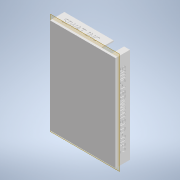
# Autodesk Inventor part: Buttom Plate
Saved by Autodesk Inventor 2020 (Build 240168000, 168)
## iProperties
Created: 2019-11-08
Part Number: Buttom Plate
Material: Generic
Document SubType Name: Modeling
Designer: siwat
Density: 1 g/cm^3
Appearance: Default
Author: siwat
Autodesk Inventor part; units mm, degrees
ref_plane "YZ Plane" through (0, 0, 0) normal (1, 0, 0) x (0, 1, 0)
ref_plane "XZ Plane" through (0, 0, 0) normal (0, 1, 0) x (-1, 0, 0)
ref_plane "XY Plane" through (0, 0, 0) normal (0, 0, 1) x (1, 0, 0)
ref_plane "Work Plane1" through (0, 0, 0) normal (0, 0, 1) x (1, 0, 0)
sketch "Sketch1" plane through (0, 0, 0) normal (0, 0, 1) x (1, 0, 0)
  line L0 (38.904, 56.6039) -> (-39.0955, 56.6039)
  line L1 (-39.0955, 56.6039) -> (-39.0955, -56.8569)
  line L2 (-39.0955, -56.8569) -> (38.904, -56.8569)
  line L3 (38.904, -56.8569) -> (38.904, 56.6039)
  line L4 (-37.4141, -55.0738) -> (37.4715, -55.0738)
  line L5 (37.4715, -55.0738) -> (37.4715, 55.1115)
  line L6 (37.4715, 55.1115) -> (-37.4141, 55.1115)
  line L7 (-37.4141, 55.1115) -> (-37.4141, -55.0738)
  point P0 (0, 0)
  constraints: 16 end point, 4 parallel, 2 horizontal, 2 perpendicular
extrude "Extrusion1" add sketch "Sketch1" along normal blind 2.0625 and the other way blind 14.525
sketch "Sketch2" plane through (0, 0, 2.0625) normal (0, 0, 1) x (1, 0, 0)
  line L0 (38.904, 56.6039) -> (-39.0955, 56.6039)
  line L1 (-39.0955, 56.6039) -> (-39.0955, -56.8569)
  line L2 (-39.0955, -56.8569) -> (38.904, -56.8569)
  line L3 (38.904, -56.8569) -> (38.904, 56.6039)
  point P0 (0, 0)
  constraints: 8 end point, 2 parallel, 1 horizontal, 1 perpendicular
extrude "Extrusion2" add sketch "Sketch2" along normal blind 0.59
sketch "Sketch3" plane through (-39.0955, -56.8569, -14.525) normal (-1, 0, 0) x (0, 0, 1)
  line L0 (14.525, 65.2907) -> (0, 65.2907)
  line L1 (0, 65.2907) -> (0, 84.283)
  line L2 (0, 84.283) -> (14.525, 84.283)
  line L3 (14.525, 84.283) -> (14.525, 65.2907)
  line L4 (0, 0) -> (0, 113.4608) projected
  point P0 (14.525, 56.8569)
  constraints: 8 end point, 2 parallel, 1 horizontal, 1 perpendicular, 1 point on line
extrude "Extrusion3" cut sketch "Sketch3" against normal up to surface (1.6814 mm away)
sketch "Sketch4" plane through (-39.0955, 56.6039, -14.525) normal (0, 1, 0) x (1, 0, 0)
  line L0 (77.9995, 0) -> (0, 0) projected
  line L1 (58.5885, -14.525) -> (71.0413, -14.525)
  line L2 (71.0413, -14.525) -> (71.0413, 0)
  line L3 (71.0413, 0) -> (58.5885, 0)
  line L4 (58.5885, 0) -> (58.5885, -14.525)
  point P0 (39.0955, -14.525)
  constraints: 8 end point, 2 parallel, 1 horizontal, 1 perpendicular, 1 point on line
extrude "Extrusion4" cut sketch "Sketch4" against normal up to surface (1.4924 mm away)
sketch "Sketch6" plane through (0, 0, 2.0625) normal (0, 0, -1) x (-1, 0, 0)
  line L0 (35.9141, -53.5738) -> (-35.9715, -53.5738)
  line L1 (-35.9715, -53.5738) -> (-35.9715, 53.6115)
  line L2 (-35.9715, 53.6115) -> (35.9141, 53.6115)
  line L3 (35.9141, 53.6115) -> (35.9141, -53.5738)
  line L4 (-37.4715, 55.1115) -> (-31.9458, 55.1115) projected
  line L5 (-37.4715, -55.0738) -> (-37.4715, 55.1115) projected
  line L6 (37.4141, -55.0738) -> (-37.4715, -55.0738) projected
  line L7 (37.4141, 8.4338) -> (37.4141, -55.0738) projected
  line L8 (37.4141, -55.0738) -> (37.4141, 55.1115) projected
  line L9 (-37.4715, 55.1115) -> (-37.4715, -55.0738) projected
  line L10 (37.4141, -55.0738) -> (-37.4715, -55.0738)
  line L11 (-37.4715, -55.0738) -> (-37.4715, 55.1115)
  line L12 (-37.4715, 55.1115) -> (37.4141, 55.1115)
  line L13 (37.4141, 55.1115) -> (37.4141, -55.0738)
  point P0 (0, 0)
  dimension "d12" = 1.5
  dimension "d13" = 1.5
  dimension "d14" = 1.5
  dimension "d15" = 1.5
  constraints: 16 end point, 4 parallel, 2 horizontal, 2 perpendicular
  measures "d12" distance between parallel lines of L2 L4
  measures "d13" distance between parallel lines of L5 L1
  measures "d14" distance between parallel lines of L6 L0
  measures "d15" distance between parallel lines of L7 L3
extrude "Extrusion6" add sketch "Sketch6" along normal up to surface (2.0625 mm away)
sketch "Sketch5" plane through (0, 0, 2.0625) normal (0, 0, -1) x (-1, 0, 0)
  circle A0 centre (33.0429, -48.5316) radius 1.6001
  circle A1 centre (11.8743, 21.7468) radius 1.6087
  circle A2 centre (-29.2374, 31.3404) radius 1.6463
  circle A3 centre (-15.7576, -8.1834) radius 1.5639
  circle A4 centre (-29.803, -47.9298) radius 1.5995
  point P0 (0, 0)
  constraints: 5 centre point
extrude "Extrusion5" add sketch "Sketch5" along normal blind 4.5
sketch "Sketch7" plane through (-39.0955, 56.6039, 2.6525) normal (0, 1, 0) x (1, 0, 0)
  line L0 (6.9784, 11.7138) -> (55.3893, 11.7138) construction
  line L1 (55.3893, 11.7138) -> (55.3893, 4.2787) construction
  line L2 (55.3893, 4.2787) -> (6.9784, 4.2787) construction
  line L3 (6.9784, 4.2787) -> (6.9784, 11.7138) construction
  spline S0 degree 2 poles (9.2953, 5.4005) (8.6333, 5.4005) (7.7046, 5.6771) (7.2946, 5.8747) knots 0 0 0 1 2 2 2
  line L4 (7.2946, 5.8747) -> (7.2946, 6.8924)
  line L5 (7.2946, 6.8924) -> (7.3538, 6.8924)
  spline S1 degree 2 poles (7.3538, 6.8924) (7.754, 6.5169) (8.7667, 6.102) (9.236, 6.102) knots 0 0 0 1 2 2 2
  spline S2 degree 2 poles (9.236, 6.102) (9.9078, 6.102) (10.5945, 6.6602) (10.5945, 7.1196) knots 0 0 0 1 2 2 2
  spline S3 degree 2 poles (10.5945, 7.1196) (10.5945, 7.4852) (10.2339, 7.9396) (9.8436, 8.0533) knots 0 0 0 1 2 2 2
  spline S4 degree 2 poles (9.8436, 8.0533) (9.562, 8.1323) (9.0927, 8.241) (8.742, 8.3299) knots 0 0 0 1 2 2 2
  spline S5 degree 2 poles (8.742, 8.3299) (8.4258, 8.4139) (7.9269, 8.6658) (7.7342, 8.8684) knots 0 0 0 1 2 2 2
  spline S6 degree 2 poles (7.7342, 8.8684) (7.5465, 9.0709) (7.339, 9.6143) (7.339, 9.97) knots 0 0 0 1 2 2 2
  spline S7 degree 2 poles (7.339, 9.97) (7.339, 10.711) (8.495, 11.7138) (9.3891, 11.7138) knots 0 0 0 1 2 2 2
  spline S8 degree 2 poles (9.3891, 11.7138) (9.9029, 11.7138) (10.8119, 11.5113) (11.2021, 11.3186) knots 0 0 0 1 2 2 2
  line L6 (11.2021, 11.3186) -> (11.2021, 10.3504)
  line L7 (11.2021, 10.3504) -> (11.1429, 10.3504)
  spline S9 degree 2 poles (11.1429, 10.3504) (10.8514, 10.6171) (9.9424, 11.0123) (9.4435, 11.0123) knots 0 0 0 1 2 2 2
  spline S10 degree 2 poles (9.4435, 11.0123) (8.8803, 11.0123) (8.1838, 10.4838) (8.1838, 10.054) knots 0 0 0 1 2 2 2
  spline S11 degree 2 poles (8.1838, 10.054) (8.1838, 9.6687) (8.5938, 9.2092) (8.9791, 9.1055) knots 0 0 0 1 2 2 2
  spline S12 degree 2 poles (8.9791, 9.1055) (9.236, 9.0363) (9.9819, 8.8585) (10.2289, 8.7844) knots 0 0 0 1 2 2 2
  spline S13 degree 2 poles (10.2289, 8.7844) (10.8563, 8.5917) (11.4393, 7.8161) (11.4393, 7.248) knots 0 0 0 1 2 2 2
  spline S14 degree 2 poles (11.4393, 7.248) (11.4393, 6.8874) (11.1478, 6.1958) (10.886, 5.9537) knots 0 0 0 1 2 2 2
  spline S15 degree 2 poles (10.886, 5.9537) (10.5945, 5.687) (9.8535, 5.4005) (9.2953, 5.4005) knots 0 0 0 1 2 2 2
  line L8 (14.3885, 5.5091) -> (12.0271, 5.5091)
  line L9 (12.0271, 5.5091) -> (12.0271, 6.1316)
  line L10 (12.0271, 6.1316) -> (12.8027, 6.1316)
  line L11 (12.8027, 6.1316) -> (12.8027, 10.9827)
  line L12 (12.8027, 10.9827) -> (12.0271, 10.9827)
  line L13 (12.0271, 10.9827) -> (12.0271, 11.6051)
  line L14 (12.0271, 11.6051) -> (14.3885, 11.6051)
  line L15 (14.3885, 11.6051) -> (14.3885, 10.9827)
  line L16 (14.3885, 10.9827) -> (13.6129, 10.9827)
  line L17 (13.6129, 10.9827) -> (13.6129, 6.1316)
  line L18 (13.6129, 6.1316) -> (14.3885, 6.1316)
  line L19 (14.3885, 6.1316) -> (14.3885, 5.5091)
  line L20 (22.2233, 11.6051) -> (20.6919, 5.5091)
  line L21 (20.6919, 5.5091) -> (19.783, 5.5091)
  line L22 (19.783, 5.5091) -> (18.543, 10.5677)
  line L23 (18.543, 10.5677) -> (17.3377, 5.5091)
  line L24 (17.3377, 5.5091) -> (16.4386, 5.5091)
  line L25 (16.4386, 5.5091) -> (14.8825, 11.6051)
  line L26 (14.8825, 11.6051) -> (15.7173, 11.6051)
  line L27 (15.7173, 11.6051) -> (16.9425, 6.5515)
  line L28 (16.9425, 6.5515) -> (18.1577, 11.6051)
  line L29 (18.1577, 11.6051) -> (18.9827, 11.6051)
  line L30 (18.9827, 11.6051) -> (20.2078, 6.4922)
  line L31 (20.2078, 6.4922) -> (21.428, 11.6051)
  line L32 (21.428, 11.6051) -> (22.2233, 11.6051)
  line L33 (22.2925, 5.5091) -> (24.3476, 11.6051)
  line L34 (24.3476, 11.6051) -> (25.3454, 11.6051)
  line L35 (25.3454, 11.6051) -> (27.4005, 5.5091)
  line L36 (27.4005, 5.5091) -> (26.5459, 5.5091)
  line L37 (26.5459, 5.5091) -> (25.9926, 7.2135)
  line L38 (25.9926, 7.2135) -> (23.6658, 7.2135)
  line L39 (23.6658, 7.2135) -> (23.1126, 5.5091)
  line L40 (23.1126, 5.5091) -> (22.2925, 5.5091)
  line L41 (25.7703, 7.9051) -> (24.8267, 10.7752)
  line L42 (24.8267, 10.7752) -> (23.8881, 7.9051)
  line L43 (23.8881, 7.9051) -> (25.7703, 7.9051)
  line L44 (29.4012, 5.5091) -> (29.4012, 10.8839)
  line L45 (29.4012, 10.8839) -> (27.356, 10.8839)
  line L46 (27.356, 10.8839) -> (27.356, 11.6051)
  line L47 (27.356, 11.6051) -> (32.2566, 11.6051)
  line L48 (32.2566, 11.6051) -> (32.2566, 10.8839)
  line L49 (32.2566, 10.8839) -> (30.2114, 10.8839)
  line L50 (30.2114, 10.8839) -> (30.2114, 5.5091)
  line L51 (30.2114, 5.5091) -> (29.4012, 5.5091)
  line L52 (37.6165, 5.5091) -> (35.2552, 5.5091)
  line L53 (35.2552, 5.5091) -> (35.2552, 6.1316)
  line L54 (35.2552, 6.1316) -> (36.0307, 6.1316)
  line L55 (36.0307, 6.1316) -> (36.0307, 10.9827)
  line L56 (36.0307, 10.9827) -> (35.2552, 10.9827)
  line L57 (35.2552, 10.9827) -> (35.2552, 11.6051)
  line L58 (35.2552, 11.6051) -> (37.6165, 11.6051)
  line L59 (37.6165, 11.6051) -> (37.6165, 10.9827)
  line L60 (37.6165, 10.9827) -> (36.8409, 10.9827)
  line L61 (36.8409, 10.9827) -> (36.8409, 6.1316)
  line L62 (36.8409, 6.1316) -> (37.6165, 6.1316)
  line L63 (37.6165, 6.1316) -> (37.6165, 5.5091)
  line L64 (42.9814, 5.5091) -> (42.0724, 5.5091)
  line L65 (42.0724, 5.5091) -> (39.3751, 10.7653)
  line L66 (39.3751, 10.7653) -> (39.3751, 5.5091)
  line L67 (39.3751, 5.5091) -> (38.6193, 5.5091)
  line L68 (38.6193, 5.5091) -> (38.6193, 11.6051)
  line L69 (38.6193, 11.6051) -> (39.7703, 11.6051)
  line L70 (39.7703, 11.6051) -> (42.2255, 6.7787)
  line L71 (42.2255, 6.7787) -> (42.2255, 11.6051)
  line L72 (42.2255, 11.6051) -> (42.9814, 11.6051)
  line L73 (42.9814, 11.6051) -> (42.9814, 5.5091)
  spline S16 degree 2 poles (46.5975, 5.4005) (46.0047, 5.4005) (45.0018, 5.8006) (44.6363, 6.2008) knots 0 0 0 1 2 2 2
  spline S17 degree 2 poles (44.6363, 6.2008) (44.2707, 6.596) (43.8706, 7.7816) (43.8706, 8.5522) knots 0 0 0 1 2 2 2
  spline S18 degree 2 poles (43.8706, 8.5522) (43.8706, 9.3179) (44.2608, 10.4541) (44.6313, 10.874) knots 0 0 0 1 2 2 2
  spline S19 degree 2 poles (44.6313, 10.874) (44.9969, 11.284) (45.9948, 11.7138) (46.6123, 11.7138) knots 0 0 0 1 2 2 2
  spline S20 degree 2 poles (46.6123, 11.7138) (46.9186, 11.7138) (47.457, 11.6249) (47.6843, 11.5557) knots 0 0 0 1 2 2 2
  spline S21 degree 2 poles (47.6843, 11.5557) (47.8819, 11.4915) (48.2919, 11.3087) (48.4944, 11.2001) knots 0 0 0 1 2 2 2
  line L74 (48.4944, 11.2001) -> (48.4944, 10.2219)
  line L75 (48.4944, 10.2219) -> (48.4302, 10.2219)
  spline S22 degree 2 poles (48.4302, 10.2219) (48.3215, 10.3207) (47.9856, 10.5974) (47.7436, 10.7308) knots 0 0 0 1 2 2 2
  spline S23 degree 2 poles (47.7436, 10.7308) (47.5114, 10.8592) (46.963, 11.0222) (46.6073, 11.0222) knots 0 0 0 1 2 2 2
  spline S24 degree 2 poles (46.6073, 11.0222) (46.2171, 11.0222) (45.5205, 10.7011) (45.2587, 10.3948) knots 0 0 0 1 2 2 2
  spline S25 degree 2 poles (45.2587, 10.3948) (45.0018, 10.0836) (44.7153, 9.1401) (44.7153, 8.5522) knots 0 0 0 1 2 2 2
  spline S26 degree 2 poles (44.7153, 8.5522) (44.7153, 7.9248) (45.0167, 7.0208) (45.2785, 6.7096) knots 0 0 0 1 2 2 2
  spline S27 degree 2 poles (45.2785, 6.7096) (45.5354, 6.4082) (46.222, 6.102) (46.6073, 6.102) knots 0 0 0 1 2 2 2
  spline S28 degree 2 poles (46.6073, 6.102) (46.9581, 6.102) (47.5558, 6.2749) (47.788, 6.4033) knots 0 0 0 1 2 2 2
  spline S29 degree 2 poles (47.788, 6.4033) (48.0103, 6.5317) (48.3413, 6.7985) (48.4352, 6.8924) knots 0 0 0 1 2 2 2
  line L76 (48.4352, 6.8924) -> (48.4944, 6.8924)
  line L77 (48.4944, 6.8924) -> (48.4944, 5.9241)
  spline S30 degree 2 poles (48.4944, 5.9241) (48.2919, 5.8302) (47.9362, 5.6573) (47.6843, 5.5783) knots 0 0 0 1 2 2 2
  spline S31 degree 2 poles (47.6843, 5.5783) (47.4175, 5.4894) (46.963, 5.4005) (46.5975, 5.4005) knots 0 0 0 1 2 2 2
  point P0 (39.0955, 2.6525)
  constraints: 2 other
extrude "Extrusion7" cut sketch "Sketch7" against normal blind 0.7
sketch "Sketch8" plane through (38.904, -56.8569, -14.525) normal (1, 0, 0) x (0, 0, -1)
  line L0 (-5.3389, 100.8282) -> (-5.3389, 55.9949) construction
  line L1 (-5.3389, 55.9949) -> (-8.4955, 55.9949) construction
  line L2 (-8.4955, 55.9949) -> (-8.4955, 100.8282) construction
  line L3 (-8.4955, 100.8282) -> (-5.3389, 100.8282) construction
  spline S0 degree 2 poles (-11.672, 98.5113) (-11.672, 99.1733) (-11.3953, 100.102) (-11.1977, 100.512) knots 0 0 0 1 2 2 2
  line L4 (-11.1977, 100.512) -> (-10.1801, 100.512)
  line L5 (-10.1801, 100.512) -> (-10.1801, 100.4528)
  spline S1 degree 2 poles (-10.1801, 100.4528) (-10.5555, 100.0526) (-10.9705, 99.0399) (-10.9705, 98.5706) knots 0 0 0 1 2 2 2
  spline S2 degree 2 poles (-10.9705, 98.5706) (-10.9705, 97.8988) (-10.4123, 97.2121) (-9.9528, 97.2121) knots 0 0 0 1 2 2 2
  spline S3 degree 2 poles (-9.9528, 97.2121) (-9.5873, 97.2121) (-9.1328, 97.5727) (-9.0192, 97.963) knots 0 0 0 1 2 2 2
  spline S4 degree 2 poles (-9.0192, 97.963) (-8.9401, 98.2446) (-8.8315, 98.7139) (-8.7425, 99.0646) knots 0 0 0 1 2 2 2
  spline S5 degree 2 poles (-8.7425, 99.0646) (-8.6586, 99.3808) (-8.4066, 99.8797) (-8.2041, 100.0724) knots 0 0 0 1 2 2 2
  spline S6 degree 2 poles (-8.2041, 100.0724) (-8.0015, 100.2601) (-7.4581, 100.4676) (-7.1024, 100.4676) knots 0 0 0 1 2 2 2
  spline S7 degree 2 poles (-7.1024, 100.4676) (-6.3614, 100.4676) (-5.3586, 99.3116) (-5.3586, 98.4175) knots 0 0 0 1 2 2 2
  spline S8 degree 2 poles (-5.3586, 98.4175) (-5.3586, 97.9037) (-5.5612, 96.9947) (-5.7538, 96.6045) knots 0 0 0 1 2 2 2
  line L6 (-5.7538, 96.6045) -> (-6.7221, 96.6045)
  line L7 (-6.7221, 96.6045) -> (-6.7221, 96.6637)
  spline S9 degree 2 poles (-6.7221, 96.6637) (-6.4553, 96.9552) (-6.0601, 97.8642) (-6.0601, 98.3631) knots 0 0 0 1 2 2 2
  spline S10 degree 2 poles (-6.0601, 98.3631) (-6.0601, 98.9263) (-6.5887, 99.6228) (-7.0185, 99.6228) knots 0 0 0 1 2 2 2
  spline S11 degree 2 poles (-7.0185, 99.6228) (-7.4038, 99.6228) (-7.8632, 99.2128) (-7.967, 98.8275) knots 0 0 0 1 2 2 2
  spline S12 degree 2 poles (-7.967, 98.8275) (-8.0361, 98.5706) (-8.214, 97.8247) (-8.2881, 97.5777) knots 0 0 0 1 2 2 2
  spline S13 degree 2 poles (-8.2881, 97.5777) (-8.4807, 96.9503) (-9.2563, 96.3673) (-9.8244, 96.3673) knots 0 0 0 1 2 2 2
  spline S14 degree 2 poles (-9.8244, 96.3673) (-10.185, 96.3673) (-10.8766, 96.6588) (-11.1187, 96.9206) knots 0 0 0 1 2 2 2
  spline S15 degree 2 poles (-11.1187, 96.9206) (-11.3855, 97.2121) (-11.672, 97.9531) (-11.672, 98.5113) knots 0 0 0 1 2 2 2
  line L8 (-11.5633, 93.4181) -> (-11.5633, 95.7795)
  line L9 (-11.5633, 95.7795) -> (-10.9409, 95.7795)
  line L10 (-10.9409, 95.7795) -> (-10.9409, 95.0039)
  line L11 (-10.9409, 95.0039) -> (-6.0897, 95.0039)
  line L12 (-6.0897, 95.0039) -> (-6.0897, 95.7795)
  line L13 (-6.0897, 95.7795) -> (-5.4673, 95.7795)
  line L14 (-5.4673, 95.7795) -> (-5.4673, 93.4181)
  line L15 (-5.4673, 93.4181) -> (-6.0897, 93.4181)
  line L16 (-6.0897, 93.4181) -> (-6.0897, 94.1937)
  line L17 (-6.0897, 94.1937) -> (-10.9409, 94.1937)
  line L18 (-10.9409, 94.1937) -> (-10.9409, 93.4181)
  line L19 (-10.9409, 93.4181) -> (-11.5633, 93.4181)
  line L20 (-11.5633, 88.0533) -> (-11.5633, 88.9622)
  line L21 (-11.5633, 88.9622) -> (-6.3071, 91.6595)
  line L22 (-6.3071, 91.6595) -> (-11.5633, 91.6595)
  line L23 (-11.5633, 91.6595) -> (-11.5633, 92.4153)
  line L24 (-11.5633, 92.4153) -> (-5.4673, 92.4153)
  line L25 (-5.4673, 92.4153) -> (-5.4673, 91.2643)
  line L26 (-5.4673, 91.2643) -> (-10.2937, 88.8091)
  line L27 (-10.2937, 88.8091) -> (-5.4673, 88.8091)
  line L28 (-5.4673, 88.8091) -> (-5.4673, 88.0533)
  line L29 (-5.4673, 88.0533) -> (-11.5633, 88.0533)
  spline S16 degree 2 poles (-11.672, 84.4372) (-11.672, 85.03) (-11.2718, 86.0328) (-10.8717, 86.3984) knots 0 0 0 1 2 2 2
  spline S17 degree 2 poles (-10.8717, 86.3984) (-10.4765, 86.7639) (-9.2909, 87.1641) (-8.5202, 87.1641) knots 0 0 0 1 2 2 2
  spline S18 degree 2 poles (-8.5202, 87.1641) (-7.7545, 87.1641) (-6.6183, 86.7738) (-6.1984, 86.4033) knots 0 0 0 1 2 2 2
  spline S19 degree 2 poles (-6.1984, 86.4033) (-5.7884, 86.0377) (-5.3586, 85.0399) (-5.3586, 84.4223) knots 0 0 0 1 2 2 2
  spline S20 degree 2 poles (-5.3586, 84.4223) (-5.3586, 84.1161) (-5.4475, 83.5776) (-5.5167, 83.3504) knots 0 0 0 1 2 2 2
  spline S21 degree 2 poles (-5.5167, 83.3504) (-5.5809, 83.1528) (-5.7637, 82.7427) (-5.8724, 82.5402) knots 0 0 0 1 2 2 2
  line L30 (-5.8724, 82.5402) -> (-6.8505, 82.5402)
  line L31 (-6.8505, 82.5402) -> (-6.8505, 82.6044)
  spline S22 degree 2 poles (-6.8505, 82.6044) (-6.7517, 82.7131) (-6.4751, 83.049) (-6.3417, 83.2911) knots 0 0 0 1 2 2 2
  spline S23 degree 2 poles (-6.3417, 83.2911) (-6.2132, 83.5233) (-6.0502, 84.0716) (-6.0502, 84.4273) knots 0 0 0 1 2 2 2
  spline S24 degree 2 poles (-6.0502, 84.4273) (-6.0502, 84.8175) (-6.3713, 85.5141) (-6.6776, 85.7759) knots 0 0 0 1 2 2 2
  spline S25 degree 2 poles (-6.6776, 85.7759) (-6.9888, 86.0328) (-7.9324, 86.3193) (-8.5202, 86.3193) knots 0 0 0 1 2 2 2
  spline S26 degree 2 poles (-8.5202, 86.3193) (-9.1476, 86.3193) (-10.0516, 86.018) (-10.3629, 85.7562) knots 0 0 0 1 2 2 2
  spline S27 degree 2 poles (-10.3629, 85.7562) (-10.6642, 85.4993) (-10.9705, 84.8126) (-10.9705, 84.4273) knots 0 0 0 1 2 2 2
  spline S28 degree 2 poles (-10.9705, 84.4273) (-10.9705, 84.0765) (-10.7976, 83.4788) (-10.6691, 83.2466) knots 0 0 0 1 2 2 2
  spline S29 degree 2 poles (-10.6691, 83.2466) (-10.5407, 83.0243) (-10.2739, 82.6933) (-10.1801, 82.5995) knots 0 0 0 1 2 2 2
  line L32 (-10.1801, 82.5995) -> (-10.1801, 82.5402)
  line L33 (-10.1801, 82.5402) -> (-11.1483, 82.5402)
  spline S30 degree 2 poles (-11.1483, 82.5402) (-11.2422, 82.7427) (-11.4151, 83.0984) (-11.4941, 83.3504) knots 0 0 0 1 2 2 2
  spline S31 degree 2 poles (-11.4941, 83.3504) (-11.5831, 83.6171) (-11.672, 84.0716) (-11.672, 84.4372) knots 0 0 0 1 2 2 2
  line L34 (-9.2662, 79.7244) -> (-9.2662, 82.0314)
  line L35 (-9.2662, 82.0314) -> (-8.5252, 82.0314)
  line L36 (-8.5252, 82.0314) -> (-8.5252, 79.7244)
  line L37 (-8.5252, 79.7244) -> (-9.2662, 79.7244)
  line L38 (-11.5633, 75.2092) -> (-11.5633, 78.7413)
  line L39 (-11.5633, 78.7413) -> (-5.4673, 78.7413)
  line L40 (-5.4673, 78.7413) -> (-5.4673, 77.9311)
  line L41 (-5.4673, 77.9311) -> (-10.8421, 77.9311)
  line L42 (-10.8421, 77.9311) -> (-10.8421, 75.2092)
  line L43 (-10.8421, 75.2092) -> (-11.5633, 75.2092)
  line L44 (-11.5633, 74.5719) -> (-5.4673, 74.5719)
  line L45 (-5.4673, 74.5719) -> (-5.4673, 70.7582)
  line L46 (-5.4673, 70.7582) -> (-6.1885, 70.7582)
  line L47 (-6.1885, 70.7582) -> (-6.1885, 73.7618)
  line L48 (-6.1885, 73.7618) -> (-7.8583, 73.7618)
  line L49 (-7.8583, 73.7618) -> (-7.8583, 70.9608)
  line L50 (-7.8583, 70.9608) -> (-8.5795, 70.9608)
  line L51 (-8.5795, 70.9608) -> (-8.5795, 73.7618)
  line L52 (-8.5795, 73.7618) -> (-10.8421, 73.7618)
  line L53 (-10.8421, 73.7618) -> (-10.8421, 70.7582)
  line L54 (-10.8421, 70.7582) -> (-11.5633, 70.7582)
  line L55 (-11.5633, 70.7582) -> (-11.5633, 74.5719)
  spline S32 degree 2 poles (-8.5202, 65.0624) (-9.3551, 65.0624) (-10.6988, 65.7391) (-11.0742, 66.3072) knots 0 0 0 1 2 2 2
  spline S33 degree 2 poles (-11.0742, 66.3072) (-11.3657, 66.7716) (-11.5633, 67.725) (-11.5633, 68.466) knots 0 0 0 1 2 2 2
  line L56 (-11.5633, 68.466) -> (-11.5633, 69.869)
  line L57 (-11.5633, 69.869) -> (-5.4673, 69.869)
  line L58 (-5.4673, 69.869) -> (-5.4673, 68.4809)
  spline S34 degree 2 poles (-5.4673, 68.4809) (-5.4673, 67.6213) (-5.7242, 66.6432) (-5.9514, 66.2974) knots 0 0 0 1 2 2 2
  spline S35 degree 2 poles (-5.9514, 66.2974) (-6.3417, 65.7095) (-7.631, 65.0624) (-8.5202, 65.0624) knots 0 0 0 1 2 2 2
  spline S36 degree 2 poles (-8.5104, 65.9071) (-7.8089, 65.9071) (-6.8159, 66.3715) (-6.5343, 66.8309) knots 0 0 0 1 2 2 2
  spline S37 degree 2 poles (-6.5343, 66.8309) (-6.3417, 67.1569) (-6.1688, 67.893) (-6.1688, 68.4413) knots 0 0 0 1 2 2 2
  line L59 (-6.1688, 68.4413) -> (-6.1688, 69.0588)
  line L60 (-6.1688, 69.0588) -> (-10.8618, 69.0588)
  line L61 (-10.8618, 69.0588) -> (-10.8618, 68.4413)
  spline S38 degree 2 poles (-10.8618, 68.4413) (-10.8618, 67.9029) (-10.6889, 67.0878) (-10.4567, 66.7568) knots 0 0 0 1 2 2 2
  spline S39 degree 2 poles (-10.4567, 66.7568) (-10.1702, 66.3319) (-9.2217, 65.9071) (-8.5104, 65.9071) knots 0 0 0 1 2 2 2
  line L62 (-5.4673, 57.351) -> (-11.5633, 58.8824)
  line L63 (-11.5633, 58.8824) -> (-11.5633, 59.7913)
  line L64 (-11.5633, 59.7913) -> (-6.5047, 61.0313)
  line L65 (-6.5047, 61.0313) -> (-11.5633, 62.2367)
  line L66 (-11.5633, 62.2367) -> (-11.5633, 63.1357)
  line L67 (-11.5633, 63.1357) -> (-5.4673, 64.6919)
  line L68 (-5.4673, 64.6919) -> (-5.4673, 63.857)
  line L69 (-5.4673, 63.857) -> (-10.5209, 62.6319)
  line L70 (-10.5209, 62.6319) -> (-5.4673, 61.4166)
  line L71 (-5.4673, 61.4166) -> (-5.4673, 60.5916)
  line L72 (-5.4673, 60.5916) -> (-10.5802, 59.3665)
  line L73 (-10.5802, 59.3665) -> (-5.4673, 58.1463)
  line L74 (-5.4673, 58.1463) -> (-5.4673, 57.351)
  line L75 (-11.5633, 51.3982) -> (-11.5633, 52.2084)
  line L76 (-11.5633, 52.2084) -> (-6.312, 52.2084)
  line L77 (-6.312, 52.2084) -> (-9.8837, 53.7991)
  line L78 (-9.8837, 53.7991) -> (-9.8837, 54.2931)
  line L79 (-9.8837, 54.2931) -> (-6.312, 55.869)
  line L80 (-6.312, 55.869) -> (-11.5633, 55.869)
  line L81 (-11.5633, 55.869) -> (-11.5633, 56.6248)
  line L82 (-11.5633, 56.6248) -> (-5.4673, 56.6248)
  line L83 (-5.4673, 56.6248) -> (-5.4673, 55.5182)
  line L84 (-5.4673, 55.5182) -> (-8.8611, 53.9967)
  line L85 (-8.8611, 53.9967) -> (-5.4673, 52.5246)
  line L86 (-5.4673, 52.5246) -> (-5.4673, 51.3982)
  line L87 (-5.4673, 51.3982) -> (-11.5633, 51.3982)
  line L88 (-11.5633, 46.883) -> (-11.5633, 49.8569)
  line L89 (-11.5633, 49.8569) -> (-10.9409, 49.8569)
  line L90 (-10.9409, 49.8569) -> (-10.9409, 48.7504)
  line L91 (-10.9409, 48.7504) -> (-6.8554, 48.7504)
  line L92 (-6.8554, 48.7504) -> (-6.8554, 49.8569)
  line L93 (-6.8554, 49.8569) -> (-6.2972, 49.8569)
  spline S40 degree 2 poles (-6.2972, 49.8569) (-6.2972, 49.2296) (-5.9415, 48.6368) (-5.4475, 48.5972) knots 0 0 0 1 2 2 2
  line L94 (-5.4475, 48.5972) -> (-5.4475, 47.9649)
  line L95 (-5.4475, 47.9649) -> (-10.9409, 47.9649)
  line L96 (-10.9409, 47.9649) -> (-10.9409, 46.883)
  line L97 (-10.9409, 46.883) -> (-11.5633, 46.883)
  spline S41 degree 2 poles (-11.672, 43.8894) (-11.672, 44.5513) (-11.3953, 45.4801) (-11.1977, 45.8901) knots 0 0 0 1 2 2 2
  line L98 (-11.1977, 45.8901) -> (-10.1801, 45.8901)
  line L99 (-10.1801, 45.8901) -> (-10.1801, 45.8308)
  spline S42 degree 2 poles (-10.1801, 45.8308) (-10.5555, 45.4307) (-10.9705, 44.418) (-10.9705, 43.9487) knots 0 0 0 1 2 2 2
  spline S43 degree 2 poles (-10.9705, 43.9487) (-10.9705, 43.2768) (-10.4123, 42.5902) (-9.9528, 42.5902) knots 0 0 0 1 2 2 2
  spline S44 degree 2 poles (-9.9528, 42.5902) (-9.5873, 42.5902) (-9.1328, 42.9508) (-9.0192, 43.341) knots 0 0 0 1 2 2 2
  spline S45 degree 2 poles (-9.0192, 43.341) (-8.9401, 43.6226) (-8.8315, 44.0919) (-8.7425, 44.4427) knots 0 0 0 1 2 2 2
  spline S46 degree 2 poles (-8.7425, 44.4427) (-8.6586, 44.7588) (-8.4066, 45.2578) (-8.2041, 45.4504) knots 0 0 0 1 2 2 2
  spline S47 degree 2 poles (-8.2041, 45.4504) (-8.0015, 45.6382) (-7.4581, 45.8456) (-7.1024, 45.8456) knots 0 0 0 1 2 2 2
  spline S48 degree 2 poles (-7.1024, 45.8456) (-6.3614, 45.8456) (-5.3586, 44.6897) (-5.3586, 43.7955) knots 0 0 0 1 2 2 2
  spline S49 degree 2 poles (-5.3586, 43.7955) (-5.3586, 43.2818) (-5.5612, 42.3728) (-5.7538, 41.9825) knots 0 0 0 1 2 2 2
  line L100 (-5.7538, 41.9825) -> (-6.7221, 41.9825)
  line L101 (-6.7221, 41.9825) -> (-6.7221, 42.0418)
  spline S50 degree 2 poles (-6.7221, 42.0418) (-6.4553, 42.3333) (-6.0601, 43.2422) (-6.0601, 43.7412) knots 0 0 0 1 2 2 2
  spline S51 degree 2 poles (-6.0601, 43.7412) (-6.0601, 44.3043) (-6.5887, 45.0009) (-7.0185, 45.0009) knots 0 0 0 1 2 2 2
  spline S52 degree 2 poles (-7.0185, 45.0009) (-7.4038, 45.0009) (-7.8632, 44.5909) (-7.967, 44.2055) knots 0 0 0 1 2 2 2
  spline S53 degree 2 poles (-7.967, 44.2055) (-8.0361, 43.9487) (-8.214, 43.2027) (-8.2881, 42.9557) knots 0 0 0 1 2 2 2
  spline S54 degree 2 poles (-8.2881, 42.9557) (-8.4807, 42.3283) (-9.2563, 41.7454) (-9.8244, 41.7454) knots 0 0 0 1 2 2 2
  spline S55 degree 2 poles (-9.8244, 41.7454) (-10.185, 41.7454) (-10.8766, 42.0369) (-11.1187, 42.2987) knots 0 0 0 1 2 2 2
  spline S56 degree 2 poles (-11.1187, 42.2987) (-11.3855, 42.5902) (-11.672, 43.3312) (-11.672, 43.8894) knots 0 0 0 1 2 2 2
  line L102 (-11.5633, 37.3883) -> (-11.5633, 40.9204)
  line L103 (-11.5633, 40.9204) -> (-5.4673, 40.9204)
  line L104 (-5.4673, 40.9204) -> (-5.4673, 40.1103)
  line L105 (-5.4673, 40.1103) -> (-10.8421, 40.1103)
  line L106 (-10.8421, 40.1103) -> (-10.8421, 37.3883)
  line L107 (-10.8421, 37.3883) -> (-11.5633, 37.3883)
  spline S57 degree 2 poles (-8.5202, 31.9444) (-9.3551, 31.9444) (-10.6988, 32.6212) (-11.0742, 33.1893) knots 0 0 0 1 2 2 2
  spline S58 degree 2 poles (-11.0742, 33.1893) (-11.3657, 33.6536) (-11.5633, 34.6071) (-11.5633, 35.3481) knots 0 0 0 1 2 2 2
  line L108 (-11.5633, 35.3481) -> (-11.5633, 36.751)
  line L109 (-11.5633, 36.751) -> (-5.4673, 36.751)
  line L110 (-5.4673, 36.751) -> (-5.4673, 35.3629)
  spline S59 degree 2 poles (-5.4673, 35.3629) (-5.4673, 34.5033) (-5.7242, 33.5252) (-5.9514, 33.1794) knots 0 0 0 1 2 2 2
  spline S60 degree 2 poles (-5.9514, 33.1794) (-6.3417, 32.5915) (-7.631, 31.9444) (-8.5202, 31.9444) knots 0 0 0 1 2 2 2
  spline S61 degree 2 poles (-8.5104, 32.7891) (-7.8089, 32.7891) (-6.8159, 33.2535) (-6.5343, 33.7129) knots 0 0 0 1 2 2 2
  spline S62 degree 2 poles (-6.5343, 33.7129) (-6.3417, 34.039) (-6.1688, 34.775) (-6.1688, 35.3234) knots 0 0 0 1 2 2 2
  line L111 (-6.1688, 35.3234) -> (-6.1688, 35.9409)
  line L112 (-6.1688, 35.9409) -> (-10.8618, 35.9409)
  line L113 (-10.8618, 35.9409) -> (-10.8618, 35.3234)
  spline S63 degree 2 poles (-10.8618, 35.3234) (-10.8618, 34.7849) (-10.6889, 33.9698) (-10.4567, 33.6388) knots 0 0 0 1 2 2 2
  spline S64 degree 2 poles (-10.4567, 33.6388) (-10.1702, 33.214) (-9.2217, 32.7891) (-8.5104, 32.7891) knots 0 0 0 1 2 2 2
  line L114 (-9.2662, 29.0051) -> (-9.2662, 31.3121)
  line L115 (-9.2662, 31.3121) -> (-8.5252, 31.3121)
  line L116 (-8.5252, 31.3121) -> (-8.5252, 29.0051)
  line L117 (-8.5252, 29.0051) -> (-9.2662, 29.0051)
  line L118 (-11.5633, 25.8978) -> (-11.5633, 28.2591)
  line L119 (-11.5633, 28.2591) -> (-10.9409, 28.2591)
  line L120 (-10.9409, 28.2591) -> (-10.9409, 27.4835)
  line L121 (-10.9409, 27.4835) -> (-6.0897, 27.4835)
  line L122 (-6.0897, 27.4835) -> (-6.0897, 28.2591)
  line L123 (-6.0897, 28.2591) -> (-5.4673, 28.2591)
  line L124 (-5.4673, 28.2591) -> (-5.4673, 25.8978)
  line L125 (-5.4673, 25.8978) -> (-6.0897, 25.8978)
  line L126 (-6.0897, 25.8978) -> (-6.0897, 26.6734)
  line L127 (-6.0897, 26.6734) -> (-10.9409, 26.6734)
  line L128 (-10.9409, 26.6734) -> (-10.9409, 25.8978)
  line L129 (-10.9409, 25.8978) -> (-11.5633, 25.8978)
  line L130 (-11.5633, 21.6148) -> (-11.5633, 24.5887)
  line L131 (-11.5633, 24.5887) -> (-10.9409, 24.5887)
  line L132 (-10.9409, 24.5887) -> (-10.9409, 23.4821)
  line L133 (-10.9409, 23.4821) -> (-6.8554, 23.4821)
  line L134 (-6.8554, 23.4821) -> (-6.8554, 24.5887)
  line L135 (-6.8554, 24.5887) -> (-6.2972, 24.5887)
  spline S65 degree 2 poles (-6.2972, 24.5887) (-6.2972, 23.9613) (-5.9415, 23.3685) (-5.4475, 23.329) knots 0 0 0 1 2 2 2
  line L136 (-5.4475, 23.329) -> (-5.4475, 22.6966)
  line L137 (-5.4475, 22.6966) -> (-10.9409, 22.6966)
  line L138 (-10.9409, 22.6966) -> (-10.9409, 21.6148)
  line L139 (-10.9409, 21.6148) -> (-11.5633, 21.6148)
  line L140 (-11.5633, 15.6028) -> (-11.5633, 16.655)
  line L141 (-11.5633, 16.655) -> (-9.1377, 18.5816)
  line L142 (-9.1377, 18.5816) -> (-9.1377, 19.5103)
  line L143 (-9.1377, 19.5103) -> (-11.5633, 19.5103)
  line L144 (-11.5633, 19.5103) -> (-11.5633, 20.3205)
  line L145 (-11.5633, 20.3205) -> (-5.4673, 20.3205)
  line L146 (-5.4673, 20.3205) -> (-5.4673, 18.7496)
  spline S66 degree 2 poles (-5.4673, 18.7496) (-5.4673, 18.2259) (-5.5809, 17.5195) (-5.7884, 17.1984) knots 0 0 0 1 2 2 2
  spline S67 degree 2 poles (-5.7884, 17.1984) (-5.9959, 16.8773) (-6.643, 16.5068) (-7.1222, 16.5068) knots 0 0 0 1 2 2 2
  spline S68 degree 2 poles (-7.1222, 16.5068) (-7.7891, 16.5068) (-8.6931, 17.1885) (-8.9105, 17.7714) knots 0 0 0 1 2 2 2
  line L147 (-8.9105, 17.7714) -> (-11.5633, 15.6028)
  spline S69 degree 2 poles (-7.1864, 17.3515) (-6.9197, 17.3515) (-6.5096, 17.5392) (-6.3763, 17.7368) knots 0 0 0 1 2 2 2
  spline S70 degree 2 poles (-6.3763, 17.7368) (-6.2626, 17.9098) (-6.1688, 18.3692) (-6.1688, 18.7051) knots 0 0 0 1 2 2 2
  line L148 (-6.1688, 18.7051) -> (-6.1688, 19.5103)
  line L149 (-6.1688, 19.5103) -> (-8.461, 19.5103)
  line L150 (-8.461, 19.5103) -> (-8.461, 18.799)
  spline S71 degree 2 poles (-8.461, 18.799) (-8.461, 18.4482) (-8.3375, 17.89) (-8.1448, 17.6973) knots 0 0 0 1 2 2 2
  spline S72 degree 2 poles (-8.1448, 17.6973) (-7.9768, 17.5195) (-7.5026, 17.3515) (-7.1864, 17.3515) knots 0 0 0 1 2 2 2
  line L151 (-11.5633, 11.5322) -> (-11.5633, 15.2915)
  line L152 (-11.5633, 15.2915) -> (-10.6988, 15.2915)
  spline S73 degree 2 poles (-10.6988, 15.2915) (-10.3184, 14.8865) (-9.612, 14.1652) (-9.2316, 13.8194) knots 0 0 0 1 2 2 2
  spline S74 degree 2 poles (-9.2316, 13.8194) (-8.4659, 13.1229) (-7.547, 12.614) (-7.058, 12.614) knots 0 0 0 1 2 2 2
  spline S75 degree 2 poles (-7.058, 12.614) (-6.8011, 12.614) (-6.4158, 12.7721) (-6.2923, 12.9154) knots 0 0 0 1 2 2 2
  spline S76 degree 2 poles (-6.2923, 12.9154) (-6.1688, 13.0586) (-6.0453, 13.4341) (-6.0453, 13.6613) knots 0 0 0 1 2 2 2
  spline S77 degree 2 poles (-6.0453, 13.6613) (-6.0453, 13.8787) (-6.154, 14.3233) (-6.2379, 14.5258) knots 0 0 0 1 2 2 2
  spline S78 degree 2 poles (-6.2379, 14.5258) (-6.3071, 14.6987) (-6.5047, 15.0198) (-6.5739, 15.1186) knots 0 0 0 1 2 2 2
  line L153 (-6.5739, 15.1186) -> (-6.5739, 15.1631)
  line L154 (-6.5739, 15.1631) -> (-5.7044, 15.1631)
  spline S79 degree 2 poles (-5.7044, 15.1631) (-5.5809, 14.9112) (-5.3389, 14.0071) (-5.3389, 13.602) knots 0 0 0 1 2 2 2
  spline S80 degree 2 poles (-5.3389, 13.602) (-5.3389, 12.7474) (-6.2429, 11.7841) (-7.0135, 11.7841) knots 0 0 0 1 2 2 2
  spline S81 degree 2 poles (-7.0135, 11.7841) (-7.3741, 11.7841) (-7.9768, 11.9521) (-8.2337, 12.1003) knots 0 0 0 1 2 2 2
  spline S82 degree 2 poles (-8.2337, 12.1003) (-8.5005, 12.2485) (-9.0241, 12.6783) (-9.2761, 12.9154) knots 0 0 0 1 2 2 2
  spline S83 degree 2 poles (-9.2761, 12.9154) (-9.696, 13.3007) (-10.595, 14.2442) (-10.8569, 14.5258) knots 0 0 0 1 2 2 2
  line L155 (-10.8569, 14.5258) -> (-10.8569, 11.5322)
  line L156 (-10.8569, 11.5322) -> (-11.5633, 11.5322)
  point P0 (-14.525, 56.8569)
  constraints: 2 other
extrude "Extrusion8" cut sketch "Sketch8" against normal blind 0.7
body "Solid1"
